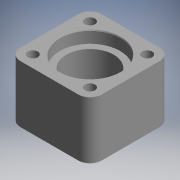
# Autodesk Inventor part: 552157 EAMK-A-D40-44A/C---(1O)
Saved by Autodesk Inventor 2017.3 (Build 213256000, 256)
## iProperties
Part Number: 552157 EAMK-A-D40-44A/C---(1O)
Material: Generic
Catalog Web Link: www.cadenas.de
Description: EAMK-A O-coupling housing
Vendor: FESTO
Document SubType Name: Modeling
Designer: partserver
Manufacturer: FESTO
Mass: 64.9553 g
Surface Area: 213.654 cm^2
Volume: 64.9553 cm^3
Density: 1 g/cm^3
Appearance: PSOLRGB-192-192-192
Category: PARTsolutions
Company: FESTO
Title: 552157 EAMK-A-D40-44A/C---(1O)
Author: Cadenas PARTsolutions
Comments: coupling housing
PSOL_IDENT_0: {$CADENAS_DATA\23d-libs\festo\parts\e\eamk\eamk_a.prj},213 {VTYP=3D},{NB=552157 EAMK-A-D40-44A/C---(
PSOL_IDENT_1: 1O)},{LINA=552157 EAMK-A-D40-44A/C---(1O)},{NN=EAMK-A O},{DATE=06.06.2021 22:52:14},{GEOMDATE=06.06.
PSOL_IDENT_2: 2021 22:51:00},{VERSION=},{LINEID=170},{WBVAR=SVERS},{WBNUMERIC=SVERS}  {NB=552157 EAMK-A-D40-44A/C-
PSOL_IDENT_3: --(1O)},{LINA=552157 EAMK-A-D40-44A/C---(1O)},{KT=DUMMY},{TNR=552157},{TYP=EAMK-A-D40-44A/C},{VERS=2
PSOL_IDENT_4: },{H3=0.0},{H4=0.0},{B1=0.00},{B2=0.000},{B3=0.0},{B4=0.000},{D1=0.0},{D2=0.0},{D3=0},{D4=0},{D4NDM=
PSOL_IDENT_5: 0.000},{D5=0},{D6=-},{D6N=0.000},{D7=-},{D7N=0.000},{D8=0},{D9=0},{D10=0},{D11=0.0},{H1=0.0},{H2=0},
PSOL_IDENT_6: {H5=0.0},{H6=0.000},{L1=0.000},{L2=0.0},{L3=0.000},{L4=0.000},{L5=0.000},{L6=0.000},{L7=0.0},{L8=0},
PSOL_IDENT_7: {L9=0},{L10=0},{L11=0},{L12=0},{L13=0.000},{SW=0.0},{RA=0.000},{RB=0.000},{RC=0.000},{SVERS=1},{R1=0
PSOL_IDENT_8: .000},{R2=0.000},{R3=0.000},{R4=0.000},{W=0.000},{W1=0.000},{H7=0.000},{CNSMASSEXACT=0.000}
NB: 552157 EAMK-A-D40-44A/C---(1O)
NN: EAMK-A O
NT: coupling housing
NBSYN: $TNR. $TYP.---($SVERS.O)
LINA: 552157 EAMK-A-D40-44A/C---(1O)
CATALOG: Festo
TNR: 552157
TYP: EAMK-A-D40-44A/C
H3: 0
H4: 0
B1: 0
B2: 0
B3: 0
B4: 0
D1: 0
D2: 0
D3: 0
D4: 0
D5: 0
D6: -
D7: -
D8: 0
D9: 0
D10: 0
D11: 0
H1: 0
H2: 0
H5: 0
H6: 0
L1: 0
L2: 0
L3: 0
L4: 0
L5: 0
L6: 0
L7: 0
L8: 0
L9: 0
L10: 0
L11: 0
L12: 0
L13: 0
SW: 0
RA: 0
RB: 0
RC: 0
SVERS: 1
R1: 0
R2: 0
R3: 0
R4: 0
W: 0
W1: 0
H7: 0
CNSMASSEXACT: 0
SUPPLIER: FESTO
ARTICLENO: 552157 EAMK-A-D40-44A/C---(1O)
BOMINFO: 552157 EAMK-A-D40-44A/C---(1O)
CREATOR: CADENAS GmbH
Autodesk Inventor part; units mm, degrees
sketch "Skizze_1" plane through (0, 0, -38) normal (0, 0, 1) x (1, 0, 0)
  line L0 (-27, 19.25) -> (-27, -19.25)
  arc A0 (-27, -19.25) -> (-19.25, -27) centre (-19.25, -19.25) ccw
  line L1 (-19.25, -27) -> (19.25, -27)
  arc A1 (19.25, -27) -> (27, -19.25) centre (19.25, -19.25) ccw
  line L2 (27, -19.25) -> (27, 19.25)
  arc A2 (27, 19.25) -> (19.25, 27) centre (19.25, 19.25) ccw
  line L3 (19.25, 27) -> (-19.25, 27)
  arc A3 (-19.25, 27) -> (-27, 19.25) centre (-19.25, 19.25) ccw
  constraints: 8 end point, 8 point on circle, 4 centre point
extrude "Extrusion1" add sketch "Skizze_1" along normal blind 38
sketch "Skizze_2" plane through (0, 0, 0) normal (1, 0, 0) x (0, 1, 0)
  line L0 (0, 0) -> (0, 3)
  line L1 (0, 3) -> (21.6536, 3)
  line L2 (21.6536, 3) -> (22, 2.4)
  line L3 (22, 2.4) -> (22, 0.3)
  arc A0 (22, 0.3) -> (22.3, 0) centre (22.3, 0.3) ccw
  line L4 (22.3, 0) -> (0, 0)
  line L5 (0, 0) -> (0, 3)
  constraints: 12 end point, 2 point on circle, 1 centre point
revolve "Revolution1" add sketch "Skizze_2" angle 360 about axis through (0, 0, 0) along (0, 0, 1)
sketch "Skizze_3" plane through (0, 0, 0) normal (1, 0, 0) x (0, 1, 0)
  line L0 (0, -38) -> (0, 3)
  line L1 (0, 3) -> (16, 3)
  line L2 (16, 3) -> (15.712, -30)
  line L3 (15.712, -30) -> (20, -30)
  line L4 (20, -30) -> (20, -37.4)
  line L5 (20, -37.4) -> (20.3464, -38)
  line L6 (20.3464, -38) -> (0, -38)
  line L7 (0, -38) -> (0, 3)
  constraints: 16 end point
revolve "Revolution2" cut sketch "Skizze_3" angle 360 about axis through (0, 0, -38) along (0, 0, 1)
sketch "Sketch4" plane through (0, 0, 3) normal (0, 0, 1) x (1, 0, 0)
  point P0 (0, 19)
hole "Hole1" at (0, 19, 3) direction (0, 0, -1) diameter 3.242 depth 15 tip angle 120 countersink diameter 4 countersink angle 90 thread size "M4x0.7" class "6H" standard "ISO Metric profile"
sketch "Sketch5" plane through (0, 0, 3) normal (0, 0, 1) x (1, 0, 0)
  point P0 (0, -19)
hole "Hole2" at (0, -19, 3) direction (0, 0, -1) diameter 3.242 depth 15 tip angle 120 countersink diameter 4 countersink angle 90 thread size "M4x0.7" class "6H" standard "ISO Metric profile"
sketch "Sketch6" plane through (0, 0, 3) normal (0, 0, 1) x (1, 0, 0)
  point P0 (19, 0)
hole "Hole3" at (19, 0, 3) direction (0, 0, -1) diameter 3.242 depth 15 tip angle 120 countersink diameter 4 countersink angle 90 thread size "M4x0.7" class "6H" standard "ISO Metric profile"
sketch "Sketch7" plane through (0, 0, 3) normal (0, 0, 1) x (1, 0, 0)
  point P0 (-19, 0)
hole "Hole4" at (-19, 0, 3) direction (0, 0, -1) diameter 3.242 depth 15 tip angle 120 countersink diameter 4 countersink angle 90 thread size "M4x0.7" class "6H" standard "ISO Metric profile"
sketch "Skizze_8" plane through (19, 0, 0) normal (1, 0, 0) x (0, 0, -1)
  line L0 (38, 19) -> (-3, 19)
  line L1 (-3, 19) -> (-3, 24.9713)
  line L2 (-3, 24.9713) -> (24, 24.5)
  line L3 (24, 24.5) -> (24, 22.3)
  line L4 (24, 22.3) -> (38, 22.3)
  line L5 (38, 22.3) -> (38, 19)
  line L6 (38, 19) -> (-3, 19)
  constraints: 14 end point
revolve "Revolution3" cut sketch "Skizze_8" angle 360 about axis through (19, 19, -38) along (0, 0, 1)
sketch "Skizze_9" plane through (19, 0, 0) normal (1, 0, 0) x (0, 0, -1)
  line L0 (38, -19) -> (-3, -19)
  line L1 (-3, -19) -> (-3, -13.0287)
  line L2 (-3, -13.0287) -> (24, -13.5)
  line L3 (24, -13.5) -> (24, -15.7)
  line L4 (24, -15.7) -> (38, -15.7)
  line L5 (38, -15.7) -> (38, -19)
  line L6 (38, -19) -> (-3, -19)
  constraints: 14 end point
revolve "Revolution4" cut sketch "Skizze_9" angle 360 about axis through (19, -19, -38) along (0, 0, 1)
sketch "Skizze_10" plane through (-19, 0, 0) normal (1, 0, 0) x (0, 0, -1)
  line L0 (38, 19) -> (-3, 19)
  line L1 (-3, 19) -> (-3, 24.9713)
  line L2 (-3, 24.9713) -> (24, 24.5)
  line L3 (24, 24.5) -> (24, 22.3)
  line L4 (24, 22.3) -> (38, 22.3)
  line L5 (38, 22.3) -> (38, 19)
  line L6 (38, 19) -> (-3, 19)
  constraints: 14 end point
revolve "Revolution5" cut sketch "Skizze_10" angle 360 about axis through (-19, 19, -38) along (0, 0, 1)
sketch "Skizze_11" plane through (-19, 0, 0) normal (1, 0, 0) x (0, 0, -1)
  line L0 (38, -19) -> (-3, -19)
  line L1 (-3, -19) -> (-3, -13.0287)
  line L2 (-3, -13.0287) -> (24, -13.5)
  line L3 (24, -13.5) -> (24, -15.7)
  line L4 (24, -15.7) -> (38, -15.7)
  line L5 (38, -15.7) -> (38, -19)
  line L6 (38, -19) -> (-3, -19)
  constraints: 14 end point
revolve "Revolution6" cut sketch "Skizze_11" angle 360 about axis through (-19, -19, -38) along (0, 0, 1)
ref_plane "ADAPTER_XY" through (0, 0, -38) normal (0, 0, 1) x (1, 0, 0)
ref_plane "ADAPTER_YZ" through (0, 0, -38) normal (1, 0, 0) x (0, 1, 0)
ref_plane "ADAPTER_ZX" through (0, 0, -38) normal (0, 1, 0) x (0, 0, 1)
ref_plane "ANBAU_XY" through (0, 0, -38) normal (0, 0, 1) x (1, 0, 0)
ref_plane "ANBAU_YZ" through (0, 0, -38) normal (1, 0, 0) x (0, 1, 0)
ref_plane "ANBAU_ZX" through (0, 0, -38) normal (0, 1, 0) x (0, 0, 1)
ref_plane "ANBAU_1_XY" through (0, 0, 3) normal (0, 0, 1) x (1, 0, 0)
ref_plane "ANBAU_1_YZ" through (0, 0, 3) normal (1, 0, 0) x (0, 1, 0)
ref_plane "ANBAU_1_ZX" through (0, 0, 3) normal (0, 1, 0) x (0, 0, 1)
ref_plane "EAMK_XY" through (0, 0, -38) normal (0, 0, 1) x (1, 0, 0)
ref_plane "EAMK_YZ" through (0, 0, -38) normal (1, 0, 0) x (0, 1, 0)
ref_plane "EAMK_ZX" through (0, 0, -38) normal (0, 1, 0) x (0, 0, 1)
ref_plane "Kupplung_XY" through (0, 0, -29.6) normal (0, 0, -1) x (1, 0, 0)
ref_plane "Kupplung_YZ" through (0, 0, -29.6) normal (1, 0, 0) x (0, -1, 0)
ref_plane "Kupplung_ZX" through (0, 0, -29.6) normal (0, -1, 0) x (0, 0, -1)
ref_plane "MOTORFLANSCH_XY" through (0, 0, 0) normal (0, 0, 1) x (1, 0, 0)
ref_plane "MOTORFLANSCH_YZ" through (0, 0, 0) normal (1, 0, 0) x (0, 1, 0)
ref_plane "MOTORFLANSCH_ZX" through (0, 0, 0) normal (0, 1, 0) x (0, 0, 1)
ref_plane "ZYL_SCHRAUBE_1_1_XY" through (-19, 19, -24) normal (0, 0, 1) x (1, 0, 0)
ref_plane "ZYL_SCHRAUBE_1_1_YZ" through (-19, 19, -24) normal (1, 0, 0) x (0, 1, 0)
ref_plane "ZYL_SCHRAUBE_1_1_ZX" through (-19, 19, -24) normal (0, 1, 0) x (0, 0, 1)
ref_plane "ZYL_SCHRAUBE_1_2_XY" through (19, 19, -24) normal (0, 0, 1) x (1, 0, 0)
ref_plane "ZYL_SCHRAUBE_1_2_YZ" through (19, 19, -24) normal (1, 0, 0) x (0, 1, 0)
ref_plane "ZYL_SCHRAUBE_1_2_ZX" through (19, 19, -24) normal (0, 1, 0) x (0, 0, 1)
ref_plane "ZYL_SCHRAUBE_1_3_XY" through (19, -19, -24) normal (0, 0, 1) x (1, 0, 0)
ref_plane "ZYL_SCHRAUBE_1_3_YZ" through (19, -19, -24) normal (1, 0, 0) x (0, 1, 0)
ref_plane "ZYL_SCHRAUBE_1_3_ZX" through (19, -19, -24) normal (0, 1, 0) x (0, 0, 1)
ref_plane "ZYL_SCHRAUBE_1_4_XY" through (-19, -19, -24) normal (0, 0, 1) x (1, 0, 0)
ref_plane "ZYL_SCHRAUBE_1_4_YZ" through (-19, -19, -24) normal (1, 0, 0) x (0, 1, 0)
ref_plane "ZYL_SCHRAUBE_1_4_ZX" through (-19, -19, -24) normal (0, 1, 0) x (0, 0, 1)
ref_plane "ZYL_SCHRAUBE_2_1_XY" through (22.2739, 22.2739, 0) normal (0, 0, 1) x (1, 0, 0)
ref_plane "ZYL_SCHRAUBE_2_1_YZ" through (22.2739, 22.2739, 0) normal (1, 0, 0) x (0, 1, 0)
ref_plane "ZYL_SCHRAUBE_2_1_ZX" through (22.2739, 22.2739, 0) normal (0, 1, 0) x (0, 0, 1)
ref_plane "ZYL_SCHRAUBE_2_2_XY" through (-22.2739, 22.2739, 0) normal (0, 0, 1) x (1, 0, 0)
ref_plane "ZYL_SCHRAUBE_2_2_YZ" through (-22.2739, 22.2739, 0) normal (1, 0, 0) x (0, 1, 0)
ref_plane "ZYL_SCHRAUBE_2_2_ZX" through (-22.2739, 22.2739, 0) normal (0, 1, 0) x (0, 0, 1)
ref_plane "ZYL_SCHRAUBE_2_3_XY" through (-22.2739, -22.2739, 0) normal (0, 0, 1) x (1, 0, 0)
ref_plane "ZYL_SCHRAUBE_2_3_YZ" through (-22.2739, -22.2739, 0) normal (1, 0, 0) x (0, 1, 0)
ref_plane "ZYL_SCHRAUBE_2_3_ZX" through (-22.2739, -22.2739, 0) normal (0, 1, 0) x (0, 0, 1)
ref_plane "ZYL_SCHRAUBE_2_4_XY" through (22.2739, -22.2739, 0) normal (0, 0, 1) x (1, 0, 0)
ref_plane "ZYL_SCHRAUBE_2_4_YZ" through (22.2739, -22.2739, 0) normal (1, 0, 0) x (0, 1, 0)
ref_plane "ZYL_SCHRAUBE_2_4_ZX" through (22.2739, -22.2739, 0) normal (0, 1, 0) x (0, 0, 1)
ref_plane "ZYL_SCHRAUBE_2x_1_XY" through (23.57, 23.57, 0) normal (0, 0, 1) x (1, 0, 0)
ref_plane "ZYL_SCHRAUBE_2x_1_YZ" through (23.57, 23.57, 0) normal (1, 0, 0) x (0, 1, 0)
ref_plane "ZYL_SCHRAUBE_2x_1_ZX" through (23.57, 23.57, 0) normal (0, 1, 0) x (0, 0, 1)
ref_plane "ZYL_SCHRAUBE_2x_2_XY" through (-23.57, 23.57, 0) normal (0, 0, 1) x (1, 0, 0)
ref_plane "ZYL_SCHRAUBE_2x_2_YZ" through (-23.57, 23.57, 0) normal (1, 0, 0) x (0, 1, 0)
ref_plane "ZYL_SCHRAUBE_2x_2_ZX" through (-23.57, 23.57, 0) normal (0, 1, 0) x (0, 0, 1)
ref_plane "ZYL_SCHRAUBE_2x_3_XY" through (-23.57, -23.57, 0) normal (0, 0, 1) x (1, 0, 0)
ref_plane "ZYL_SCHRAUBE_2x_3_YZ" through (-23.57, -23.57, 0) normal (1, 0, 0) x (0, 1, 0)
ref_plane "ZYL_SCHRAUBE_2x_3_ZX" through (-23.57, -23.57, 0) normal (0, 1, 0) x (0, 0, 1)
ref_plane "ZYL_SCHRAUBE_2x_4_XY" through (23.57, -23.57, 0) normal (0, 0, 1) x (1, 0, 0)
ref_plane "ZYL_SCHRAUBE_2x_4_YZ" through (23.57, -23.57, 0) normal (1, 0, 0) x (0, 1, 0)
ref_plane "ZYL_SCHRAUBE_2x_4_ZX" through (23.57, -23.57, 0) normal (0, 1, 0) x (0, 0, 1)
ref_plane "ZYL_SCHRAUBE_3_1_XY" through (19, 0, 4.7) normal (0, 0, 1) x (1, 0, 0)
ref_plane "ZYL_SCHRAUBE_3_1_YZ" through (19, 0, 4.7) normal (1, 0, 0) x (0, 1, 0)
ref_plane "ZYL_SCHRAUBE_3_1_ZX" through (19, 0, 4.7) normal (0, 1, 0) x (0, 0, 1)
ref_plane "ZYL_SCHRAUBE_3_2_XY" through (0, -19, 4.7) normal (0, 0, 1) x (1, 0, 0)
ref_plane "ZYL_SCHRAUBE_3_2_YZ" through (0, -19, 4.7) normal (1, 0, 0) x (0, 1, 0)
ref_plane "ZYL_SCHRAUBE_3_2_ZX" through (0, -19, 4.7) normal (0, 1, 0) x (0, 0, 1)
ref_plane "ZYL_SCHRAUBE_3_3_XY" through (-19, 0, 4.7) normal (0, 0, 1) x (1, 0, 0)
ref_plane "ZYL_SCHRAUBE_3_3_YZ" through (-19, 0, 4.7) normal (1, 0, 0) x (0, 1, 0)
ref_plane "ZYL_SCHRAUBE_3_3_ZX" through (-19, 0, 4.7) normal (0, 1, 0) x (0, 0, 1)
ref_plane "to_eamf_XY" through (0, 0, 0.5) normal (0, 0, 1) x (1, 0, 0)
ref_plane "to_eamf_YZ" through (0, 0, 0.5) normal (1, 0, 0) x (0, 1, 0)
ref_plane "to_eamf_ZX" through (0, 0, 0.5) normal (0, 1, 0) x (0, 0, 1)
body "Solid1"
